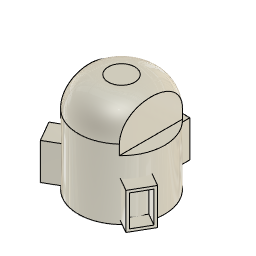
Arm Assembly v7 (Autodesk Fusion 360 archive; units mm, degrees)
design "GripperBase"
Autodesk Fusion 360 part; units mm, degrees
note: some values were not read from the file. Chosen so that the rebuilt part matches the saved one: which face or edge a step refers to.
cylinder "CylinderPrimitive1" add diameter 130 height 90 placed x (1, 0, 0) y (0, 1, 0) z (0, 0, 1) at (0, 0, 0) makes body 1
sketch "Sketch2" plane through (0, 0, 90) normal (0, 0, 1) x (-1, 0, 0)
  circle A0 centre (0, 0) radius 65
  line L0 (-48.333, 90.1713) -> (48.333, 90.1713)
  line L1 (48.333, 90.1713) -> (48.333, -90.1713)
  line L2 (48.333, -90.1713) -> (-48.333, -90.1713)
  line L3 (-48.333, -90.1713) -> (-48.333, 90.1713)
  line L4 (-48.333, 90.1713) -> (48.333, -90.1713) construction
  line L5 (48.333, 90.1713) -> (-48.333, -90.1713) construction
  dimension "d3" = 96.666
  constraint horizontal L0
  constraint perpendicular L0 L1
  constraint parallel L0 L2
  constraint parallel L1 L3
  constraint coincident L4 A0.centre
  constraint coincident L5 A0.centre
  constraint coincident A0.centre origin
  measures "d3" distance of L1.end L2.end
extrude "Extrude1" add sketch "Sketch2" along normal blind 60 contours A0 L1 L3 bodies 1
fillet "Fillet1" radius 45 2 edges at (0, -65, 150) (0, 65, 150) on bodies 1
sketch "Sketch3" plane through (0, 0, 0) normal (0, 1, 0) x (1, 0, 0)
  line L0 (-100, -50) -> (-135, -50)
  line L1 (-135, -50) -> (-135, 5)
  line L2 (-135, 5) -> (-100, 5)
  line L3 (-100, 5) -> (-100, -50)
  dimension "d8" = 35
  dimension "d9" = 55
  constraint horizontal L0
  constraint vertical L1
  constraint horizontal L2
  constraint vertical L3
  measures "d8" distance of L0.start L0.end
  measures "d9" distance of L0.start L2.end
extrude "Extrude2" add sketch "Sketch3" along normal blind 25 separate body makes body 2
shell "Shell1" thickness 4 removed faces 1 at (-123.3333, 25, 31.6667) on bodies 2
move_body "Move1" bodies 2 to x (1, 0, 0) y (0, 1, 0) z (0, 0, 1) at (120, 100, 0)
move_body "Move2" bodies 2 to x (1, 0, 0) y (0, 1, 0) z (0, 0, 1) at (0, -40, 10)
move_body "Move3" bodies 2 to x (1, 0, 0) y (0, 1, 0) z (0, 0, 1) at (-2, 0, 0)
pattern_circular "C-Pattern1" count 3 over 360 about axis through (0, 0, 1.75) along (0, 0, 1) of bodies 2 makes body 3 at (-49.2949, -34.6188, 41.6667) makes body 4 at (54.6282, -25.3812, 41.6667)
sketch "Sketch4" plane through (0, 0, 0) normal (1, 0, 0) x (0, 1, 0)
  spline S0 degree 5 poles (120, 50) (120.9439, 49.7089) (122.795, 48.8856) (125.462, 46.9265) (128.7962, 42.8574) (132.5527, 35.3492) (135.7794, 25.5812) (138.2923, 13.8408) (139.8777, 0.4417) (140.32, -14.3417) (139.4402, -30.3579) (137.1167, -47.6205) (133.2605, -66.2635) (127.8044, -86.5136) (120.6927, -108.6541) (111.8765, -132.9888) (103.4257, -154.4384) (96.2865, -171.7372) (91.1689, -183.8206) (88.5206, -190) knots 0 0 0 0 0 0 0.066667 0.133333 0.2 0.266667 0.333333 0.4 0.466667 0.533333 0.6 0.666667 0.733333 0.8 0.866667 0.933333 1 1 1 1 1 1
  line L0 (88.5206, -190) -> (85.5947, -167.6213)
  line L1 (85.5947, -167.6213) -> (90, -150)
  spline S1 degree 5 poles (90, -150) (89.6943, -151.2226) (89.3837, -152.7881) (89.8193, -152.4981) (91.9668, -147.3896) (96.1074, -135.8839) (100.7484, -121.6327) (105.28, -106.2838) (109.3228, -90.9928) (112.7001, -76.4645) (115.377, -63.0677) (117.418, -50.9107) (118.9386, -39.9283) (120.0617, -29.9587) (120.873, -20.8216) (121.376, -12.394) (121.5159, -4.6004) (121.2034, 2.6002) (120.339, 9.2255) (118.8361, 15.2823) (116.6484, 20.7797) (114.3384, 24.7382) (112.2911, 27.4634) (110.7869, 29.1725) (110, 30) knots 0 0 0 0 0 0 0.05 0.1 0.15 0.2 0.25 0.3 0.35 0.4 0.45 0.5 0.55 0.6 0.65 0.7 0.75 0.8 0.85 0.9 0.95 1 1 1 1 1 1
  line L2 (110, 30) -> (120, 50)
  line L3 (103.5206, -155) -> (73.5206, -225)
  line L4 (94.4053, -132.3787) -> (85.5947, -167.6213)
  point P0 (130, 40)
  point P1 (140, -10)
  point P2 (93.4596, -143.0809)
  point P3 (120, -30)
  point P4 (120, 10)
  constraint midpoint S0.end L3
  constraint midpoint L1.end L4
  constraint coincident L0.end L1.start
  constraint parallel L1 L4
sketch "Sketch5" plane through (48.333, 0, 0) normal (1, 0, 0) x (0, 1, 0)
  spline S0 degree 3 poles (-43.4617, 105) (-43.4617, 106.4851) (-43.3444, 108.1111) (-42.8362, 111.3202) (-42.4456, 112.9033) (-41.4968, 115.8437) (-40.8303, 117.4738) (-39.2244, 120.5945) (-38.2854, 122.0853) (-36.1741, 124.9697) (-34.753, 126.5971) (-31.6286, 129.5579) (-29.9265, 130.8924) (-27.1649, 132.7533) (-25.8853, 133.5258) (-23.2482, 134.9249) (-21.8909, 135.5521) (-17.5623, 137.3326) (-14.0739, 138.358) (-6.9524, 139.6691) (-3.3203, 139.9606) (3.3203, 139.9606) (6.9524, 139.6691) (14.0739, 138.358) (17.5623, 137.3326) (21.8909, 135.5521) (23.2482, 134.9249) (25.8853, 133.5258) (27.1649, 132.7533) (29.9265, 130.8924) (31.6286, 129.5579) (34.753, 126.5971) (36.1741, 124.9697) (38.2854, 122.0853) (39.2244, 120.5945) (40.8303, 117.4738) (41.4968, 115.8437) (42.4456, 112.9033) (42.8362, 111.3202) (43.3444, 108.1111) (43.4617, 106.4851) (43.4617, 105) knots 5.844045 5.844045 5.844045 5.844045 6.289563 6.289563 6.735082 6.735082 7.216466 7.216466 7.69785 7.69785 8.288831 8.288831 8.879813 8.879813 9.287855 9.287855 9.695897 9.695897 10.691994 10.691994 11.68809 11.68809 12.684187 12.684187 13.680283 13.680283 14.088326 14.088326 14.496368 14.496368 15.087349 15.087349 15.678331 15.678331 16.159715 16.159715 16.641099 16.641099 17.086617 17.086617 17.532136 17.532136 17.532136 17.532136
  line L0 (-43.4617, 105) -> (-43.4617, 90)
  line L1 (-43.4617, 90) -> (43.4617, 90)
  line L2 (43.4617, 90) -> (43.4617, 105)
  line L3 (0, 90) -> (-120, 90)
  line L4 (-120, 90) -> (-120, 180)
  line L5 (-120, 180) -> (100, 180)
  line L6 (100, 180) -> (100, 90)
  line L7 (100, 90) -> (-30, 90)
  constraint midpoint L1 L3.start
  constraint parallel L1 L3
  constraint perpendicular L1 L4
  constraint perpendicular L4 L5
  constraint perpendicular L5 L6
  constraint coincident L1 L7.end
  constraint perpendicular L2 L7
extrude "Extrude4" cut sketch "Sketch5" against normal blind 4 bodies 1
scale "Scale1" factor 0.4 about (-48.333, -43.4617, 105) bodies 1 3 2 4
scale "Scale2" factor 1.4 about (-9.6295, -43.7268, 66.6) bodies 1 2 3 4

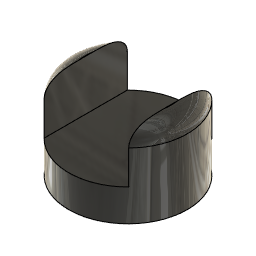
design "arm_base"
Autodesk Fusion 360 part; units mm, degrees
cylinder "CylinderPrimitive1" add diameter 130 height 90 placed x (1, 0, 0) y (0, 1, 0) z (0, 0, 1) at (0, 0, 0)
sketch "Sketch2" plane through (0, 0, 90) normal (0, 0, 1) x (-1, 0, 0)
  circle A0 centre (0, 0) radius 65
  line L0 (-46.3335, 70.1365) -> (46.3335, 70.1365)
  line L1 (46.3335, 70.1365) -> (46.3335, -70.1365)
  line L2 (46.3335, -70.1365) -> (-46.3335, -70.1365)
  line L3 (-46.3335, -70.1365) -> (-46.3335, 70.1365)
  line L4 (-46.3335, 70.1365) -> (46.3335, -70.1365) construction
  line L5 (46.3335, 70.1365) -> (-46.3335, -70.1365) construction
  constraint horizontal L0
  constraint perpendicular L0 L1
  constraint parallel L0 L2
  constraint parallel L1 L3
  constraint coincident L4 A0.centre
  constraint coincident L5 A0.centre
  constraint coincident A0.centre origin
extrude "Extrude1" cut sketch "Sketch2" against normal blind 55 contours A0 L1 L3
sketch "Sketch4" plane through (0, 0, 35) normal (0, 0, -1) x (1, 0, 0)
sketch "Sketch6" plane through (0, 0, 0) normal (0, 0, -1) x (1, 0, 0)
  circle A0 centre (-175, 0) radius 60
  line L0 (-221.333, 107.0842) -> (-128.667, 107.0842)
  line L1 (-128.667, 107.0842) -> (-128.667, -107.0842)
  line L2 (-128.667, -107.0842) -> (-221.333, -107.0842)
  line L3 (-221.333, -107.0842) -> (-221.333, 107.0842)
  line L4 (-221.333, 107.0842) -> (-128.667, -107.0842) construction
  line L5 (-128.667, 107.0842) -> (-221.333, -107.0842) construction
  point P0 (-175, 0)
  dimension "d9" = 92.666
  constraint horizontal L0
  constraint perpendicular L0 L1
  constraint parallel L0 L2
  constraint parallel L1 L3
  constraint coincident L4 P0
  constraint coincident L5 P0
  constraint coincident P0 A0.centre
  measures "d9" distance of L1.end L2.end
fillet "Fillet1" radius 18 3 edges at (60.1526, 24.6305, 90) (-65, 0, 90) (60.1526, -24.6305, 90)
scale "Scale1" factor 0.4 about (-46.3335, -7.8873, 90) bodies 1
scale "Scale2" factor 1.4 about (-46.3335, -1.5775, 90) bodies 1
